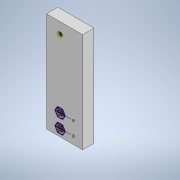
# Autodesk Inventor part: jenga
Saved by Autodesk Inventor 2020 (Build 240168000, 168)
## iProperties
Created: 2022-07-20
Part Number: jenga
Material: 일반
Document SubType Name: Modeling
Designer: SeungJin
Density: 1 g/cm^3
Appearance: 기본값
Author: SeungJin
Autodesk Inventor part; units mm, degrees
ref_plane "YZ Plane" through (0, 0, 0) normal (1, 0, 0) x (0, 1, 0)
ref_plane "XZ Plane" through (0, 0, 0) normal (0, 1, 0) x (-1, 0, 0)
ref_plane "XY Plane" through (0, 0, 0) normal (0, 0, 1) x (1, 0, 0)
ref_plane "작업 평면1" through (-228, 28.5399, 10) normal (0, 0, -1) x (0, 1, 0)
sketch "스케치1" plane through (0, 0, 0) normal (0, 0, 1) x (1, 0, 0)
  circle A0 centre (-55, -18.5) radius 2.0092
  circle A1 centre (-55, -6.5) radius 2.0092
  line L0 (-35, 63.5399) -> (-35, 28.5399)
  line L1 (-67, 63.5399) -> (-35, 63.5399)
  line L2 (-67, 28.5399) -> (-67, 63.5399)
  circle A2 centre (-55, 53.5399) radius 2.1
  line L3 (0, -25) -> (-70, -25)
  line L4 (-67, 63.5399) -> (-35, 63.5399)
  line L5 (-35, 63.5399) -> (-35, -25)
  line L6 (-35, -25) -> (-67, -25)
  line L7 (-67, -25) -> (-67, 63.5399)
  point P0 (0, 0)
extrude "돌출1" add sketch "스케치1" along normal up to surface (10 mm away) contours A0 | A1 | L0 L5 L3 L7 L2 L1 | A2
sketch "스케치2" plane through (-67, 63.5399, 10) normal (0, 0, 1) x (1, 0, 0)
  circle A0 centre (12, -82.0399) radius 2.0092
  circle A1 centre (12, -10) radius 2.1 projected
  circle A2 centre (12, -70.0399) radius 2.0092
  circle A3 centre (12, -70.0399) radius 4
  circle A4 centre (12, -82.0399) radius 4
  line L0 (14.3094, -66.0399) -> (16.6188, -70.0399)
  line L1 (16.6188, -70.0399) -> (14.3094, -74.0399)
  line L2 (14.3094, -74.0399) -> (9.6906, -74.0399)
  line L3 (9.6906, -74.0399) -> (7.3812, -70.0399)
  line L4 (7.3812, -70.0399) -> (9.6906, -66.0399)
  line L5 (9.6906, -66.0399) -> (14.3094, -66.0399)
  line L6 (14.3094, -78.0399) -> (16.6188, -82.0399)
  line L7 (16.6188, -82.0399) -> (14.3094, -86.0399)
  line L8 (14.3094, -86.0399) -> (9.6906, -86.0399)
  line L9 (9.6906, -86.0399) -> (7.3812, -82.0399)
  line L10 (7.3812, -82.0399) -> (9.6906, -78.0399)
  line L11 (9.6906, -78.0399) -> (14.3094, -78.0399)
  point P0 (67, -63.5399)
  point P1 (12, -66.0399)
  point P2 (12, -78.0399)
  dimension "d2" = 8
  dimension "d3" = 8
  constraints: 24 end point, 4 coincident, 2 centre point, 2 midpoint, 2 vertical alignment, 32 other
extrude "돌출2" cut sketch "스케치2" against normal blind 5 contours A0 | A2 | A3 | A3 L0 L1 | A3 L5 L0 | L1 L2 A3 | A3 L4 L5 | L2 L3 A3 | A3 L3 L4 | A4 | A4 L6 L7 | A4 L11 L6 | L7 L8 A4 | A4 L10 L11 | L8 L9 A4 | A4 L9 L10
sketch "스케치3" plane through (-67, 63.5399, 5) normal (0, 0, 1) x (1, 0, 0)
  line L0 (9.6906, -66.0399) -> (14.3094, -66.0399) projected
  line L1 (7.3812, -70.0399) -> (9.6906, -66.0399) projected
  line L2 (9.6906, -74.0399) -> (7.3812, -70.0399) projected
  line L3 (14.3094, -74.0399) -> (9.6906, -74.0399) projected
  line L4 (16.6188, -70.0399) -> (14.3094, -74.0399) projected
  line L5 (14.3094, -66.0399) -> (16.6188, -70.0399) projected
  line L6 (16.6188, -82.0399) -> (14.3094, -86.0399) projected
  line L7 (14.3094, -78.0399) -> (16.6188, -82.0399) projected
  line L8 (9.6906, -78.0399) -> (14.3094, -78.0399) projected
  line L9 (7.3812, -82.0399) -> (9.6906, -78.0399) projected
  line L10 (9.6906, -86.0399) -> (7.3812, -82.0399) projected
  line L11 (14.3094, -86.0399) -> (9.6906, -86.0399) projected
  point P0 (67, -63.5399)
  point P1 (12, -70.0399)
  point P2 (12, -82.0399)
hole "구멍1" at (-55, -6.5, 5) at (-55, -18.5, 5) direction (0, 0, -1) diameter 5.5 end through all clearance for "Hex Head Cap Screw ISO 24017" size "M5" standard "ISO"
sketch "스케치4" plane through (0, 0, 0) normal (0, 0, -1) x (-1, 0, 0)
  circle A0 centre (55, 53.5399) radius 2.1 projected
  circle A1 centre (55, 53.5399) radius 3.6
  line L0 (58.6, 51.4615) -> (55, 49.383)
  line L1 (55, 49.383) -> (51.4, 51.4615)
  line L2 (51.4, 51.4615) -> (51.4, 55.6184)
  line L3 (51.4, 55.6184) -> (55, 57.6968)
  line L4 (55, 57.6968) -> (58.6, 55.6184)
  line L5 (58.6, 55.6184) -> (58.6, 51.4615)
  point P0 (0, 0)
  point P1 (58.6, 53.5399)
  dimension "d13" = 7.2
  constraints: 12 end point, 2 coincident, 1 horizontal alignment, 1 midpoint, 15 other
extrude "돌출3" cut sketch "스케치4" against normal blind 5 contours A0 | A1 | L5 L0 A1 | A1 L4 L5 | A1 L3 L4 | L0 L1 A1 | A1 L2 L3 | L1 L2 A1
sketch "스케치6" plane through (0, 0, 5) normal (0, 0, -1) x (-1, 0, 0)
  line L0 (51.4, 51.4615) -> (51.4, 55.6184) projected
  line L1 (55, 49.383) -> (51.4, 51.4615) projected
  line L2 (58.6, 51.4615) -> (55, 49.383) projected
  line L3 (58.6, 55.6184) -> (58.6, 51.4615) projected
  line L4 (55, 57.6968) -> (58.6, 55.6184) projected
  line L5 (51.4, 55.6184) -> (55, 57.6968) projected
  point P0 (0, 0)
  point P1 (55, 53.5399)
hole "구멍2" at (-55, 53.5399, 5) direction (0, 0, 1) diameter 4.5 end through all clearance for "Hex Head Cap Screw ISO 24017" size "M4" standard "ISO"
